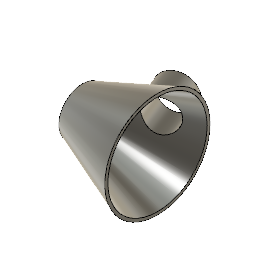
Speaker_Pneumotach_V2 (Autodesk Fusion 360 design; units mm, degrees)
Autodesk Fusion 360 part; units mm, degrees
note: some values were not read from the file. Chosen so that the rebuilt part matches the saved one: where a step ends.
sketch "Sketch3" plane through (0, 0, 0) normal (0, 0, 1) x (1, 0, 0)
  line L0 (4.9717, 32.9899) -> (4.9717, -33.0101) construction
  line L1 (-42.08, 14.7985) -> (-42.08, -14.8015) construction
  line L2 (-42.08, -14.8015) -> (4.9717, -33.0101)
  line L3 (-42.08, 14.7985) -> (4.9717, 32.9899)
  line L4 (-42.08, 14.7985) -> (-42.08, 12.8485)
  line L5 (4.9717, 32.9899) -> (4.9717, 31.0399)
  line L6 (-42.08, 12.8485) -> (4.9717, 31.0399)
  dimension "d34" = 66
  dimension "d35" = 29.6
  dimension "d37" = 1.95
  dimension "d38" = 1.95
  constraint vertical L0
  constraint vertical L1
  constraint parallel L1 L4
  constraint parallel L0 L5
  measures "d34" distance of L0.start L0.end
  measures "d35" distance of L1.start L1.end
  measures "d37" distance of L1.start L4.end
  measures "d38" distance of L0.start L5.end
revolve "Revolve1" add sketch "Sketch3" angle 360 about axis through (1.75, 0, 0) along (1, 0, 0)
ref_plane "WorkPlane1" through (-18.5542, 23.8942, 0) normal (-0.360612, 0.932716, 0) x (0, 0, -1)
sketch "Sketch10" plane through (-18.5542, 23.8942, 0) normal (-0.360612, 0.932716, 0) x (0, 0, -1)
  circle A0 centre (-0.4729, -2.4593) radius 12
  dimension "d55" = 24
  measures "d55" diameter of A0
extrude "Extrude3" add sketch "Sketch10" along normal blind 15 and the other way up to near side of body 1
hole "Hole1" at (-21.6695, 38.7718, 0.4729) direction (0.360612, -0.932716, 0) diameter 20.5 depth 25 tip angle 180
ref_plane "WorkPlane5" through (-18.5542, -23.8942, 0) normal (-0.360612, -0.932716, 0) x (0, 0, 1)
sketch "Sketch11" plane through (-18.5542, -23.8942, 0) normal (-0.360612, -0.932716, 0) x (0, 0, 1)
ref_plane "WorkPlane6" through (-18.5542, -23.8942, 0) normal (-0.360612, -0.932716, 0) x (0, 0, 1)
sketch "Sketch12" plane through (-18.5542, -23.8942, 0) normal (-0.360612, -0.932716, 0) x (0, 0, 1)
  circle A0 centre (0, -9) radius 9.978
